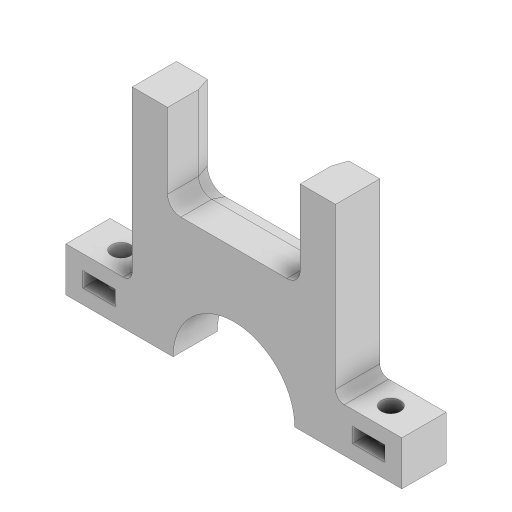
# Autodesk Inventor part: Part2
Saved by Autodesk Inventor 2023.3 (Build 273359000, 359)
## iProperties
Created: 2025-06-02
Part Number: Part2
Material: Generic
Document SubType Name: Modeling
Designer: David Zindović
Density: 1 g/cm^3
Appearance: Default
Author: David Zindović
Autodesk Inventor part; units mm, degrees
ref_plane "YZ Plane" through (0, 0, 0) normal (1, 0, 0) x (0, 1, 0)
ref_plane "XZ Plane" through (0, 0, 0) normal (0, 1, 0) x (-1, 0, 0)
ref_plane "XY Plane" through (0, 0, 0) normal (0, 0, 1) x (1, 0, 0)
sketch "Sketch1" plane through (0, 0, 0) normal (0, 0, 1) x (1, 0, 0)
  arc A0 (0, 13.75) -> (0, -13.75) centre (0, 0) ccw
  line L0 (-18.75, 0) -> (-38, 0)
  line L1 (-38, 0) -> (-38, 10)
  line L2 (-38, 10) -> (-18.75, 10)
  line L3 (-18.75, 10) -> (-18.75, 0)
  line L4 (-18.75, 0) -> (-13.75, 0)
  line L5 (-13.75, 0) -> (-13.75, 5)
  line L6 (-13.75, 5) -> (-18.75, 5)
  line L7 (-18.75, 5) -> (-18.75, 0)
  line L8 (-15, 28.25) -> (0, 28.25)
  line L9 (0, 18.75) -> (-15, 18.75)
  line L10 (-15, 18.75) -> (-15, 28.25)
  line L11 (-15, 18.75) -> (-15, 10)
  line L12 (-38, 10) -> (-31.25, 10)
  line L13 (-28.375, 0) -> (-43.75, 0)
  line L14 (-15, 10) -> (-23, 10)
  line L15 (-23, 10) -> (-23, 48.25)
  line L16 (-23, 48.25) -> (-15, 48.25)
  line L17 (-15, 48.25) -> (-15, 10)
  line L18 (-34.15, 6.7) -> (-26.85, 6.7)
  line L19 (-26.85, 6.7) -> (-26.85, 3.3)
  line L20 (-26.85, 3.3) -> (-34.15, 3.3)
  line L21 (-34.15, 3.3) -> (-34.15, 6.7)
  line L22 (0, -18.75) -> (0, 28.25)
  arc A1 (0, 18.75) -> (0, -18.75) centre (0, 0) ccw
  line L23 (-41.25, 10) -> (-31.25, 10)
  point P0 (-19, 48.25)
  point P1 (-34.15, 5)
  point P2 (-38, 5)
  point P3 (-30.5, 6.7)
  point P4 (-15, 28.25)
  point P5 (-23, 10)
  dimension "d0" = 27.5
  dimension "d3" = 10
  dimension "d10" = 20
  dimension "d12" = 7.3
  dimension "d13" = 3.4
  dimension "d14" = 8
  dimension "d16" = 5
  dimension "d17" = 5
  dimension "d18" = 15
  dimension "d19" = 5
  dimension "d20" = 15
  dimension "d21" = 9.5
  dimension "d36" = 7.5
  dimension "d42" = 15
  constraints: 48 end point, 10 parallel, 7 horizontal, 5 midpoint, 5 perpendicular, 5 point on circle, 5 point on line, 2 centre point, 2 horizontal alignment, 2 vertical alignment, 1 coincident, 1 tangent, 1 vertical
  measures "d0" diameter of A0
  measures "d3" distance of L0.end L1.end
  measures "d10" distance from line of point (-19, 48.25) L8
  measures "d12" distance of L19.end L20.end
  measures "d13" distance of L18.end L19.end
  measures "d14" distance of L15.end L16.end
  measures "d16" distance between parallel lines of L4 L6
  measures "d17" distance from line of L3 L5.end
  measures "d18" distance between parallel lines of L17 L22
  measures "d19" radial gap between concentric circles of A1 A0
  measures "d20" distance of L8.start L8.end
  measures "d21" distance between parallel lines of L9 L8
  measures "d36" distance from line of L1 point (-30.5, 6.7)
  measures "d42" distance between parallel lines of L1 L15
extrude "Extrusion1" add sketch "Sketch1" along normal blind 10 contours A0 L5 L6 A1 L14 L11 L22 | L4 A1 L6 L5 | A1 L11 L9 | L9 L10 L8 L22 | L0 L1 L2 L3 | L3 L6 A1 | L11 A1 L14 L2 L15 L16 L17 L10 | L11 L14 A1 | L3 L14 A1 L6
sketch "Sketch2" plane through (-38, 0, 0) normal (0, -1, 0) x (1, 0, 0)
  circle A0 centre (7.5, 5) radius 2.15
  line L0 (0, 0) -> (0, 10) projected
  line L1 (0, 0) -> (24.25, 0) projected
  point P0 (38, 0)
  dimension "d26" = 4.3
  dimension "d27" = 7.5
  dimension "d28" = 5
  constraints: 1 centre point
  measures "d26" diameter of A0
  measures "d27" distance from line of L0 A0.centre
  measures "d28" distance from line of L1 A0.centre
extrude "Extrusion2" cut sketch "Sketch2" against normal up to surface (10 mm away)
sketch "Sketch3" plane through (-34.15, 6.7, 0) normal (0, -1, 0) x (1, 0, 0)
  circle A0 centre (3.65, 5) radius 2.15 projected
  line L0 (0, 0) -> (7.3, 0) projected
  line L1 (7.3, 0) -> (7.3, 10) projected
  line L2 (0, 10) -> (7.3, 10) projected
  line L3 (0, 0) -> (0, 10) projected
  line L4 (3.65, 9.0415) -> (7.15, 7.0207)
  line L5 (7.15, 7.0207) -> (7.15, 2.9793)
  line L6 (7.3, 3.0659) -> (3.65, 0.9585)
  line L7 (3.65, 0.9585) -> (0, 3.0659)
  line L8 (0.15, 2.9793) -> (0.15, 7.0207)
  line L9 (0.15, 7.0207) -> (3.65, 9.0415)
  point P0 (34.15, 0)
  point P1 (7, 2.9793)
  point P2 (0, 2.9793)
  dimension "d31" = 7
  dimension "d33" = 0.9586
  constraints: 12 end point, 4 point on line, 1 coincident, 13 other
  measures "d31" distance between parallel lines of L8 L5
  measures "d33" distance from line of L0 L6.end
extrude "Extrusion3" add sketch "Sketch3" along normal up to surface (3.4 mm away) contours L3 L7 L6 L1 L0
fillet "Fillet1" radius 2 1 edges at (-23, 10, 5)
fillet "Fillet2" radius 3 1 edges at (-15, 28.25, 5)
chamfer "Chamfer1" distance 1 distance2 3 3 edges at (-6, 28.25, 0) (-14.1213, 29.1287, 0) (-15, 39.75, 0) measured on face at (-14.4749, 28.7751, 0) measured on face at (-6, 27.75, 0) measured on face at (-15.5, 39.75, 0)
mirror "Mirror1" about plane through (0, 13.75, 0) normal (1, 0, 0)
equation "\"d20\" = d18"
body "Solid1"
